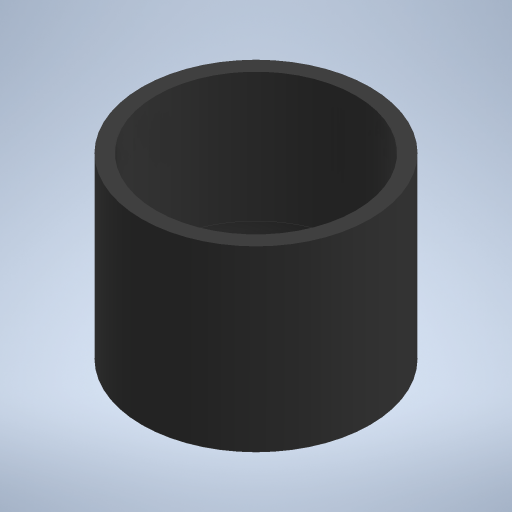
# Autodesk Inventor part: ruedas_traseras
Saved by Autodesk Inventor 2024 (Build 280153020, 153B)
## iProperties
Created: 2023-05-22
Part Number: ruedas_traseras
Material: Generic
Document SubType Name: Modeling
Designer: Diego
Density: 1 g/cm^3
Appearance: Default
Author: Diego
Autodesk Inventor part; units mm, degrees
ref_plane "YZ Plane" through (0, 0, 0) normal (1, 0, 0) x (0, 1, 0)
ref_plane "XZ Plane" through (0, 0, 0) normal (0, 1, 0) x (-1, 0, 0)
ref_plane "XY Plane" through (0, 0, 0) normal (0, 0, 1) x (1, 0, 0)
sketch "Sketch1" plane through (0, 0, 0) normal (1, 0, 0) x (0, 1, 0)
  line L0 (0, 0) -> (1.5, 0) construction
  line L1 (0, 0) -> (1.5, 0)
  line L2 (1.5, 0) -> (1.5, -10)
  line L3 (0, 0) -> (0, -16)
  arc A0 (1.5, -10) -> (6.8525, -14) centre (6.4031, -9.0202) ccw
  line L4 (0, 0) -> (25, 0) construction
  line L5 (0, -16) -> (25, -16)
  line L6 (6.8525, -14) -> (25, -14)
  line L7 (25, -14) -> (25, -16)
  dimension "d2" = 1.5
  dimension "d6" = 10
  dimension "d8" = 16
  dimension "d20" = 25
  dimension "d21" = 2
  dimension "d22" = 5
  constraints: 16 end point, 3 horizontal, 2 perpendicular, 2 point on circle, 1 centre point, 1 collinear, 1 vertical
  measures "d2" distance of L0.start L0.end
  measures "d6" distance of L0.end L2.end
  measures "d8" distance of L0.start L3.end
  measures "d20" distance of L0.start L4.end
  measures "d21" distance of L6.end L5.end
  measures "d22" radius of A0
revolve "Revolution1" add sketch "Sketch1" angle 180 about axis through (0, 0, 0) along (0, 1, 0) and the other way 180
sketch "Sketch3" plane through (0, 0, 0) normal (0, -1, 0) x (1, 0, 0)
  circle A0 centre (0, 0) radius 2.4
  dimension "d25" = 4.8
  constraints: 1 centre point, 1 coincident
  measures "d25" diameter of A0
extrude "Extrusion1" cut sketch "Sketch3" against normal blind 10
body "Solid1"
